battery (Autodesk Fusion 360 design; units mm, degrees)
Autodesk Fusion 360 part; units mm, degrees
sketch "Sketch1" plane through (0, 0, 0) normal (0, 1, 0) x (1, 0, 0)
  line L0 (0, 0) -> (-55, 0)
  line L1 (-55, 0) -> (-55, -35)
  line L2 (-55, -35) -> (0, -35)
  line L3 (0, -35) -> (0, 0)
  dimension "d1" = 55
  dimension "d2" = 35
  constraint horizontal L0
  constraint vertical L1
  constraint horizontal L2
  constraint vertical L3
  constraint coincident L0.start L3.end
  measures "d1" distance of L1.end L2.end
  measures "d2" distance of L0.end L1.end
extrude "Extrude1" add sketch "Sketch1" along normal blind 11.5
sketch "Sketch2" plane through (0, 0, 35) normal (0, 0, 1) x (-1, 0, 0)
  line L0 (55, 0) -> (0, 0)
  line L1 (0, 0) -> (0, -11.5)
  line L2 (0, -11.5) -> (55, -11.5)
  line L3 (55, -11.5) -> (55, 0)
  line L4 (55, -9.75) -> (45, -9.75)
  line L5 (45, -9.75) -> (45, -1.75)
  line L6 (45, -1.75) -> (55, -1.75)
  line L7 (55, -1.75) -> (55, -9.75)
  line L8 (45, -5.75) -> (55, -5.75)
  dimension "d5" = 10
  dimension "d6" = 8
  constraint horizontal L4
  constraint vertical L5
  constraint horizontal L6
  constraint vertical L7
  constraint coincident L3 L4.start
  constraint midpoint L5 L8.start
  constraint midpoint L7 L8.end
  constraint midpoint L3 L8.end
  measures "d5" distance of L4.start L4.end
  measures "d6" distance of L4.end L5.end
extrude "Extrude2" add sketch "Sketch2" along normal blind 4 contours L3 L5 L6 L7 L8 | L3 L4 L5 L7 L8
